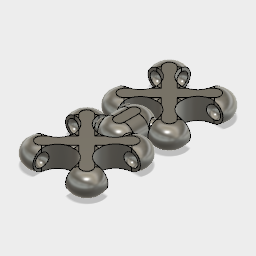
Modular_components (Autodesk Fusion 360 design; units mm, degrees)
Autodesk Fusion 360 part; units mm, degrees
box "BoxPrimitive1" add length 10 width 29.8 height 6.5 placed x (0, 0, 1) y (1, 0, 0) z (0, 1, 0) at (0, 0, 0) makes body 1
fillet "Fillet1" radius 5 4 edges at (29.8, 3.25, 10) (29.8, 3.25, 0) (0, 3.25, 10) (0, 3.25, 0) on bodies 1
fillet "Fillet3" radius 3.25 8 edges at (14.9, 6.5, 0) (29.8, 6.5, 5) (14.9, 6.5, 10) (0, 6.5, 5) (14.9, 0, 0) (0, 0, 5) (14.9, 0, 10) (29.8, 0, 5) on bodies 1
copy_body "CopyPasteBodies1" bodies 1 makes body 2
move_body "Move1" bodies 2 to x (0, 0, -1) y (0, 1, 0) z (1, 0, 0) at (9.9, 0, 19.9)
box "BoxPrimitive2" add length 20 width 10 height 6.5 placed x (0, 0, 1) y (1, 0, 0) z (0, 1, 0) at (50, 0, 0) separate body makes body 3
fillet "Fillet2" radius 5 4 edges at (50, 3.25, 0) (60, 3.25, 0) (60, 3.25, 20) (50, 3.25, 20) on bodies 3
sphere "SpherePrimitive1" add diameter 4 placed x (1, 0, 0) y (0, 0, -1) z (0, 1, 0) at (30, 0, 30) separate body makes body 4
move_body "MoveFace1" bodies 4 to x (1, 0, 0) y (0, 1, 0) z (0, 0, 1) at (20, 3.25, -25) on bodies 4
copy_body "CopyPasteBodies2" bodies 4 makes body 5
move_body "Move3" bodies 5 to x (1, 0, 0) y (0, 1, 0) z (0, 0, 1) at (10, 0, 0)
combine "Combine1" operation add target body 4 tool bodies 5 3
pattern_circular "C-Pattern1" count 4 over 360 about axis through (55, 0, 5) along (0, 1, 0) of bodies 4 makes body 6 at (61.667, 6.5, 6.6667) makes body 7 at (60, 3.2002, -2.3321) makes body 8 at (48.333, 6.5, 3.3333)
move_body "Move4" bodies 4 6 7 8 to x (1, 0, 0) y (0, 1, 0) z (0, 0, 1) at (21, 0, 0)
move_body "Move10" bodies 7 to x (1, 0, 0) y (0, 1, 0) z (0, 0, 1) at (0, 0, -28)
move_body "Move11" bodies 8 to x (1, 0, 0) y (0, 1, 0) z (0, 0, 1) at (-28, 0, 0)
move_body "Move12" bodies 8 6 to x (1, 0, 0) y (0, 1, 0) z (0, 0, 1) at (13, 0, -15)
move_body "Move13" bodies 4 7 to x (1, 0, 0) y (0, 1, 0) z (0, 0, 1) at (-1, 0, 0)
move_body "Move14" bodies 8 6 to x (1, 0, 0) y (0, 1, 0) z (0, 0, 1) at (0, 0, 1)
combine "Combine2" operation add target body 2 tool bodies 1
copy_body "CopyPasteBodies3" bodies 2 makes body 9
move_body "Move15" bodies 9 to x (0.707107, 0, 0.707107) y (0, 1, 0) z (-0.707107, 0, 0.707107) at (67.8996, 0, -23.0714)
move_body "Move16" bodies 4 to x (1, 0, 0) y (0, 1, 0) z (0, 0, 1) at (-0.125, 0, -5)
move_body "Move17" bodies 7 to x (1, 0, 0) y (0, 1, 0) z (0, 0, 1) at (0, 0, 5)
move_body "Move18" bodies 6 to x (1, 0, 0) y (0, 1, 0) z (0, 0, 1) at (-5.25, 0, 0)
move_body "Move19" bodies 8 to x (1, 0, 0) y (0, 1, 0) z (0, 0, 1) at (5, 0, 0)
move_body "Move9" bodies 7 to x (1, 0, 0) y (0, 1, 0) z (0, 0, 1) at (-0.125, 0, 0.2)
move_body "Move5" bodies 8 to x (1, 0, 0) y (0, 1, 0) z (0, 0, 1) at (-10, 0, 0)
move_body "Move20" bodies 8 to x (1, 0, 0) y (0, 1, 0) z (0, 0, 1) at (10, 0, 0)
combine "Combine3" operation cut target body 9 tool bodies 4 6 8 7 keep tools
move_body "Move21" bodies 9 to x (1, 0, 0) y (0, 1, 0) z (0, 0, 1) at (0, 0, 45)
sketch "Sketch6" plane through (0, 0, 0) normal (0, 1, 0) x (1, 0, 0)
  line L0 (0, -40) -> (4, -40)
  line L1 (4, -40) -> (4, -51.5)
  line L2 (4, -51.5) -> (0, -51.5)
  line L3 (0, -51.5) -> (0, -40)
  dimension "d23" = 4
  dimension "d24" = 11.5
  measures "d23" distance of L0.start L0.end
  measures "d24" distance of L0.start L2.end
sphere "SpherePrimitive2" add diameter 4.2 placed x (1, 0, 0) y (0, 0, -1) z (0, 1, 0) at (2, 0, 42) separate body makes body 10
copy_body "CopyPasteBodies5" bodies 10 makes body 11
move_body "Move25" bodies 11 to x (1, 0, 0) y (0, 1, 0) z (0, 0, 1) at (0, 0, 7.5)
copy_body "CopyPasteBodies6" bodies 11 10 makes body 12 makes body 13
move_body "Move26" bodies 12 13 to x (1, 0, 0) y (0, 1, 0) z (0, 0, 1) at (7.5, 0, 0)
box "BoxPrimitive3" add length 14 width 9.5 height 6.5 placed x (0, 0, 1) y (1, 0, 0) z (0, 1, 0) at (20, 0, 40) separate body makes body 14
fillet "Fillet5" radius 4.75 4 edges at (29.5, 3.25, 54) (20, 3.25, 54) (20, 3.25, 40) (29.5, 3.25, 40) on bodies 14
fillet "Fillet6" radius 3.25 8 edges at (29.5, 6.5, 47) (24.75, 6.5, 54) (20, 6.5, 47) (24.75, 6.5, 40) (20, 0, 47) (24.75, 0, 54) (29.5, 0, 47) (24.75, 0, 40) on bodies 14
move_body "Move27" bodies 14 to x (1, 0, 0) y (0, 1, 0) z (0, 0, 1) at (-19, -3, -1)
move_body "Move28" bodies 13 10 12 11 to x (1, 0, 0) y (0, 1, 0) z (0, 0, 1) at (0, 0.25, 0)
combine "Combine5" operation add target body 14 tool bodies 10 12 13 11 keep tools
move_body "Move29" bodies 14 to x (1, 0, 0) y (0, 1, 0) z (0, 0, 1) at (69, 3.5, 10)
copy_body "CopyPasteBodies7" bodies 9 makes body 15
move_body "Move30" bodies 15 to x (1, 0, 0) y (0, 1, 0) z (0, 0, 1) at (0, 0, 25)
move_body "Move31" bodies 14 to x (1, 0, 0) y (0, 1, 0) z (0, 0, 1) at (0, 0, -7)
move_body "Move32" bodies 15 to x (1, 0, 0) y (0, 1, 0) z (0, 0, 1) at (0, 0, 0.5)
hidden bodies 2 4 6 8 7 10 11 12 13
